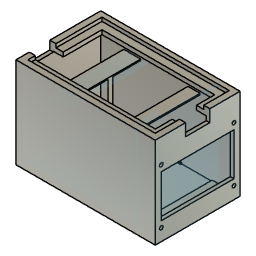
new_research_control v1 (Autodesk Fusion 360 design; units mm, degrees)
Autodesk Fusion 360 part; units mm, degrees
sketch "Sketch1" plane through (0, 0, 0) normal (0, 0, 1) x (1, 0, 0)
  line L0 (0, 0) -> (100, 0)
  line L1 (100, 0) -> (100, 70)
  line L2 (100, 70) -> (0, 70)
  line L3 (0, 70) -> (0, 0)
  constraint horizontal L0
  constraint vertical L1
  constraint horizontal L2
  constraint vertical L3
  constraint coincident L0.start L3.end
extrude "Extrude1" add sketch "Sketch1" along normal blind 75
shell "Shell1" thickness 3 removed faces 0 bodies 1
sketch "Sketch2" plane through (0, 0, 75) normal (0, 0, 1) x (-1, 0, 0)
  line L0 (0, -70) -> (0, 0)
  line L1 (0, 0) -> (-100, 0)
  line L2 (-100, 0) -> (-100, -70)
  line L3 (-100, -70) -> (0, -70)
  line L4 (-95, -5) -> (-5, -5)
  line L5 (-5, -5) -> (-5, -66)
  line L6 (-5, -66) -> (-95, -66)
  line L7 (-95, -66) -> (-95, -5)
  constraint horizontal L4
  constraint vertical L5
  constraint horizontal L6
  constraint vertical L7
extrude "Extrude2" cut sketch "Sketch2" against normal blind 73 contours L4 L5 L6 L7
sketch "Sketch3" plane through (97, 0, 0) normal (-1, 0, 0) x (0, -1, 0)
  line L0 (-67, 3) -> (-3, 3)
  line L1 (-3, 3) -> (-3, 72)
  line L2 (-3, 72) -> (-67, 72)
  line L3 (-67, 72) -> (-67, 3)
  line L4 (-67, 72) -> (-3, 72)
  line L5 (-3, 72) -> (-3, 68)
  line L6 (-3, 68) -> (-67, 68)
  line L7 (-67, 68) -> (-67, 72)
  constraint horizontal L4
  constraint vertical L5
  constraint horizontal L6
  constraint vertical L7
  constraint coincident L1 L5.end
  constraint coincident L2.end L3.start
sketch "Sketch4" plane through (0, 0, 0) normal (-1, 0, 0) x (0, -1, 0)
  line L0 (-70, 0) -> (0, 0)
  line L1 (0, 0) -> (0, 75)
  line L2 (0, 75) -> (-70, 75)
  line L3 (-70, 75) -> (-70, 0)
  line L4 (-8, 75) -> (-28, 75)
  line L5 (-28, 75) -> (-28, 68)
  line L6 (-28, 68) -> (-8, 68)
  line L7 (-8, 68) -> (-8, 75)
  constraint horizontal L4
  constraint vertical L5
  constraint horizontal L6
  constraint vertical L7
  constraint coincident L2 L4.start
extrude "Extrude3" cut sketch "Sketch4" against normal blind 24 contours L2 L4 L5 L6 L7
sketch "Sketch5" plane through (100, 0, 0) normal (1, 0, 0) x (0, 1, 0)
  line L0 (0, 0) -> (70, 0)
  line L1 (70, 0) -> (70, 75)
  line L2 (70, 75) -> (0, 75)
  line L3 (0, 75) -> (0, 0)
sketch "Sketch6" plane through (100, 0, 0) normal (1, 0, 0) x (0, 1, 0)
  line L0 (25, 75) -> (45, 75)
  line L1 (45, 75) -> (45, 63)
  line L2 (45, 63) -> (25, 63)
  line L3 (25, 63) -> (25, 75)
  constraint horizontal L0
  constraint vertical L1
  constraint horizontal L2
  constraint vertical L3
extrude "Extrude4" cut sketch "Sketch6" against normal blind 20
sketch "Sketch7" plane through (0, 3, 0) normal (0, 1, 0) x (-1, 0, 0)
  line L0 (-97, 3) -> (-3, 3)
  line L1 (-3, 3) -> (-3, 72)
  line L2 (-3, 72) -> (-97, 72)
  line L3 (-97, 72) -> (-97, 3)
sketch "Sketch8" plane through (0, 3, 0) normal (0, 1, 0) x (-1, 0, 0)
sketch "Sketch9" plane through (0, 3, 0) normal (0, 1, 0) x (-1, 0, 0)
sketch "Sketch10" plane through (97, 0, 0) normal (-1, 0, 0) x (0, -1, 0)
  line L0 (-45, 63) -> (-45, 72)
  line L1 (-45, 72) -> (-67, 72)
  line L2 (-67, 72) -> (-67, 3)
  line L3 (-67, 3) -> (-3, 3)
  line L4 (-3, 3) -> (-3, 72)
  line L5 (-3, 72) -> (-25, 72)
  line L6 (-25, 72) -> (-25, 63)
  line L7 (-25, 63) -> (-45, 63)
  line L8 (-25, 72) -> (-3, 72)
  line L9 (-3, 72) -> (-3, 68.5)
  line L10 (-3, 68.5) -> (-25, 68.5)
  line L11 (-25, 68.5) -> (-25, 72)
  constraint horizontal L8
  constraint vertical L9
  constraint horizontal L10
  constraint vertical L11
  constraint coincident L4 L9.end
  constraint coincident L5.end L6.start
sketch "Sketch11" plane through (97, 0, 0) normal (-1, 0, 0) x (0, -1, 0)
extrude "Extrude5" add sketch "Sketch10" along normal blind 5 contours L4 L5 L6 L8 L9 L10 L11
sketch "Sketch12" plane through (92, 0, 0) normal (-1, 0, 0) x (0, -1, 0)
  line L0 (-25, 68.5) -> (-3, 68.5)
  line L1 (-3, 68.5) -> (-3, 72)
  line L2 (-3, 72) -> (-5, 72)
  line L3 (-5, 72) -> (-25, 72)
  line L4 (-25, 72) -> (-25, 68.5)
sketch "Sketch13" plane through (92, 0, 0) normal (-1, 0, 0) x (0, -1, 0)
  line L0 (-3, 68.5) -> (-8, 68.5)
  line L1 (-8, 68.5) -> (-8, 72)
  line L2 (-8, 72) -> (-3, 72)
  line L3 (-3, 72) -> (-3, 68.5)
  constraint horizontal L0
  constraint vertical L1
  constraint horizontal L2
  constraint vertical L3
extrude "Extrude6" add sketch "Sketch13" along normal blind 89
move_face "MoveFace1" by (0, 45, 0) 1 faces at (99, 25, 68.8333)
sketch "Sketch14" plane through (100, 0, 0) normal (1, 0, 0) x (0, 1, 0)
  line L0 (25, 75) -> (40, 75)
  line L1 (40, 75) -> (40, 65)
  line L2 (40, 65) -> (25, 65)
  line L3 (25, 65) -> (25, 75)
  constraint horizontal L0
  constraint vertical L1
  constraint horizontal L2
  constraint vertical L3
extrude "Extrude7" cut sketch "Sketch14" against normal blind 20
extrude "Extrude8" cut 1 faces at (97.3333, 40, 71.8333) along direction (0, 1, 0) blind 5
sketch "Sketch15" plane through (92, 0, 0) normal (-1, 0, 0) x (0, -1, 0)
  line L0 (-45, 68.5) -> (-45, 72)
  line L1 (-45, 72) -> (-66, 72)
  line L2 (-66, 72) -> (-67, 72)
  line L3 (-67, 72) -> (-67, 68.5)
  line L4 (-67, 68.5) -> (-45, 68.5)
  line L5 (-67, 68.5) -> (-63, 68.5)
  line L6 (-63, 68.5) -> (-63, 72)
  line L7 (-63, 72) -> (-67, 72)
  line L8 (-67, 72) -> (-67, 68.5)
  constraint horizontal L5
  constraint vertical L6
  constraint horizontal L7
  constraint vertical L8
  constraint coincident L1 L6.end
  constraint coincident L3.end L4.start
extrude "Extrude9" add sketch "Sketch15" along normal blind 91 contours L1 L2 L3 L4 L5 L6 L7 L8
sketch "Sketch16" plane through (0, 63, 0) normal (0, -1, 0) x (1, 0, 0)
  line L0 (3, 72) -> (3, 68.5)
  line L1 (3, 68.5) -> (92, 68.5)
  line L2 (92, 68.5) -> (92, 72)
  line L3 (92, 72) -> (5, 72)
  line L4 (5, 72) -> (3, 72)
  line L5 (3, 68.5) -> (8, 68.5)
  line L6 (8, 68.5) -> (8, 72)
  line L7 (8, 72) -> (3, 72)
  line L8 (3, 72) -> (3, 68.5)
  constraint horizontal L5
  constraint vertical L6
  constraint horizontal L7
  constraint vertical L8
  constraint coincident L3 L6.end
  constraint coincident L0.end L1.start
extrude "Extrude10" add sketch "Sketch16" along normal blind 35 contours L0 L1 L3 L4 L5 L6 L7 L8
sketch "Sketch17" plane through (0, 67, 0) normal (0, -1, 0) x (1, 0, 0)
  line L0 (97, 68.5) -> (3, 68.5)
  line L1 (3, 68.5) -> (3, 3)
  line L2 (3, 3) -> (97, 3)
  line L3 (97, 3) -> (97, 68.5)
  line L4 (25, 60) -> (85, 60)
  line L5 (85, 60) -> (85, 59)
  line L6 (85, 59) -> (25, 59)
  line L7 (25, 59) -> (25, 60)
  constraint horizontal L4
  constraint vertical L5
  constraint horizontal L6
  constraint vertical L7
extrude "Extrude11" add sketch "Sketch17" along normal blind 65 contours L4 L5 L6 L7
sketch "Sketch18" plane through (0, 0, 60) normal (0, 0, 1) x (-1, 0, 0)
  line L0 (-25, -3) -> (-85, -3)
  line L1 (-85, -3) -> (-85, -67)
  line L2 (-85, -67) -> (-25, -67)
  line L3 (-25, -67) -> (-25, -3)
  line L4 (-42, -67) -> (-75, -67)
  line L5 (-75, -67) -> (-75, -3)
  line L6 (-75, -3) -> (-42, -3)
  line L7 (-42, -3) -> (-42, -67)
  constraint horizontal L4
  constraint vertical L5
  constraint horizontal L6
  constraint vertical L7
  constraint coincident L0 L5.end
  constraint coincident L2 L4.start
extrude "Extrude12" cut sketch "Sketch18" against normal blind 8 contours L0 L2 L4 L5 L6 L7
sketch "Sketch19" plane through (0, 70, 0) normal (0, 1, 0) x (-1, 0, 0)
  line L0 (-100, 75) -> (-100, 0)
  line L1 (-100, 0) -> (0, 0)
  line L2 (0, 0) -> (0, 75)
  line L3 (0, 75) -> (-100, 75)
  line L4 (-95, 2) -> (-70, 2)
  line L5 (-70, 2) -> (-70, 23)
  line L6 (-70, 23) -> (-95, 23)
  line L7 (-95, 23) -> (-95, 2)
  constraint horizontal L4
  constraint vertical L5
  constraint horizontal L6
  constraint vertical L7
extrude "Extrude13" cut sketch "Sketch19" against normal blind 11 contours L4 L5 L6 L7
sketch "Sketch20" plane through (97, 0, 0) normal (-1, 0, 0) x (0, -1, 0)
  line L0 (-25, 65) -> (-45, 65)
  line L1 (-45, 65) -> (-45, 68.5)
  line L2 (-45, 68.5) -> (-67, 68.5)
  line L3 (-67, 68.5) -> (-67, 3)
  line L4 (-67, 3) -> (-3, 3)
  line L5 (-3, 3) -> (-3, 68.5)
  line L6 (-3, 68.5) -> (-25, 68.5)
  line L7 (-25, 68.5) -> (-25, 65)
  line L8 (-58, 19) -> (-55, 19)
  line L9 (-55, 19) -> (-55, 16)
  line L10 (-55, 16) -> (-58, 16)
  line L11 (-58, 16) -> (-58, 19)
  constraint horizontal L8
  constraint vertical L9
  constraint horizontal L10
  constraint vertical L11
extrude "Extrude14" add sketch "Sketch20" along normal blind 97 contours L8 L9 L10 L11
sketch "Sketch21" plane through (0, 0, 60) normal (0, 0, 1) x (-1, 0, 0)
  line L0 (-42, -3) -> (-42, -67)
  line L1 (-42, -67) -> (-25, -67)
  line L2 (-25, -67) -> (-25, -3)
  line L3 (-25, -3) -> (-42, -3)
extrude "Extrude15" add 1 faces at (25, 24.3333, 59.3333) along direction (-1, 0, 0) blind 3
sketch "Sketch22" plane through (0, 0, 60) normal (0, 0, 1) x (-1, 0, 0)
  line L0 (-36, -13) -> (-29, -13)
  line L1 (-29, -13) -> (-29, -18)
  line L2 (-29, -18) -> (-36, -18)
  line L3 (-36, -18) -> (-36, -13)
  constraint horizontal L0
  constraint vertical L1
  constraint horizontal L2
  constraint vertical L3
extrude "Extrude16" add sketch "Sketch22" against normal blind 58
sketch "Sketch23" plane through (0, 0, 60) normal (0, 0, 1) x (-1, 0, 0)
  line L0 (-36, -40) -> (-30, -40)
  line L1 (-30, -40) -> (-30, -44)
  line L2 (-30, -44) -> (-36, -44)
  line L3 (-36, -44) -> (-36, -40)
  constraint horizontal L0
  constraint vertical L1
  constraint horizontal L2
  constraint vertical L3
extrude "Extrude17" add sketch "Sketch23" against normal blind 58
delete_face "DeleteFace1" 1 faces at (65.6667, 57, 19)
extrude "Extrude18" add 1 faces at (78.3333, 69, 23) along direction (0, 0, -1) blind 21
sketch "Sketch24" plane through (100, 0, 0) normal (1, 0, 0) x (0, 1, 0)
  line L0 (5, 50) -> (65, 50)
  line L1 (65, 50) -> (65, 15)
  line L2 (65, 15) -> (5, 15)
  line L3 (5, 15) -> (5, 50)
  constraint horizontal L0
  constraint vertical L1
  constraint horizontal L2
  constraint vertical L3
extrude "Extrude19" cut sketch "Sketch24" against normal blind 7
sketch "Sketch25" plane through (100, 0, 0) normal (1, 0, 0) x (0, 1, 0)
  line L0 (5, 50) -> (5, 55)
  line L1 (65, 50) -> (65, 55)
  constraint vertical L0
  constraint parallel L0 L1
hole "Hole1" at (100, 5, 55) direction (-1, 0, 0) diameter 3 depth 21 tip angle 118
sketch "Sketch26" plane through (100, 0, 0) normal (1, 0, 0) x (0, 1, 0)
  line L0 (65, 50) -> (65, 55)
  constraint vertical L0
hole "Hole2" at (100, 65, 55) direction (-1, 0, 0) diameter 3 depth 21 tip angle 118
sketch "Sketch27" plane through (100, 0, 0) normal (1, 0, 0) x (0, 1, 0)
  line L0 (5, 15) -> (5, 10)
  constraint vertical L0
hole "Hole3" at (100, 5, 10) direction (-1, 0, 0) diameter 3 depth 20 tip angle 118
sketch "Sketch28" plane through (100, 0, 0) normal (1, 0, 0) x (0, 1, 0)
  line L0 (65, 15) -> (65, 10)
  constraint vertical L0
hole "Hole4" at (100, 65, 10) direction (-1, 0, 0) diameter 3 depth 20 tip angle 118
extrude "Extrude20" add 1 faces at (33.3333, 8, 69.6667) along direction (0, 1, 0) blind 3
move_face "MoveFace2" by (-3, 0, 0) 1 faces at (92, 15.6667, 70.8333)
move_face "MoveFace3" by (-3, 0, 0) 1 faces at (92, 57, 70.8333)
move_face "MoveFace4" by (0, -3, 0) 1 faces at (35, 63, 69.6667)
move_face "MoveFace5" by (3, 0, 0) 1 faces at (8, 38.6667, 69.6667)
sketch "Sketch29" plane through (0, 0, 2) normal (0, 0, 1) x (-1, 0, 0)
  line L0 (-95, -67) -> (-70, -67)
  line L1 (-70, -67) -> (-70, -66)
  line L2 (-70, -66) -> (-5, -66)
  line L3 (-5, -66) -> (-5, -5)
  line L4 (-5, -5) -> (-95, -5)
  line L5 (-95, -5) -> (-95, -67)
  line L6 (-29, -13) -> (-29, -18)
  line L7 (-29, -18) -> (-36, -18)
  line L8 (-36, -18) -> (-36, -13)
  line L9 (-36, -13) -> (-29, -13)
  line L10 (-30, -40) -> (-30, -44)
  line L11 (-30, -44) -> (-36, -44)
  line L12 (-36, -44) -> (-36, -40)
  line L13 (-36, -40) -> (-30, -40)
move_face "MoveFace6" by (15, 0, 0) 6 faces at (89, 55, 70.8333) (95, 52, 73) (97, 31.6667, 55) (89, 15.6667, 70.8333) (95, 18.3333, 74) (100, 31.6667, 55)
extrude "Extrude21" cut 1 faces at (42, 45.6667, 59.6667) along direction (-1, 0, 0) blind 6
sketch "Sketch30" plane through (115, 0, 0) normal (1, 0, 0) x (0, 1, 0)
  circle A0 centre (65, 10) radius 1.5
  circle A1 centre (5, 10) radius 1.5
  circle A2 centre (65, 55) radius 1.5
  circle A3 centre (5, 55) radius 1.5
  line L0 (65, 50) -> (65, 15)
  line L1 (65, 15) -> (5, 15)
  line L2 (5, 15) -> (5, 50)
  line L3 (5, 50) -> (65, 50)
  line L4 (45, 65) -> (25, 65)
  line L5 (25, 65) -> (25, 75)
  line L6 (25, 75) -> (0, 75)
  line L7 (0, 75) -> (0, 0)
  line L8 (0, 0) -> (70, 0)
  line L9 (70, 0) -> (70, 75)
  line L10 (70, 75) -> (45, 75)
  line L11 (45, 75) -> (45, 65)
sketch "Sketch31" plane through (0, 0, 60) normal (0, 0, 1) x (-1, 0, 0)
sketch "Sketch32" plane through (115, 0, 0) normal (1, 0, 0) x (0, 1, 0)
sketch "Sketch33" plane through (115, 0, 0) normal (1, 0, 0) x (0, 1, 0)
